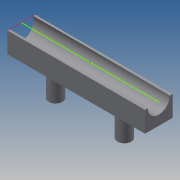
# Autodesk Inventor part: 滑軌2
Saved by Autodesk Inventor 2015 (Build 190159000, 159)
## iProperties
Created: 2018-01-06
Part Number: 滑軌2
Material: 一般
Document SubType Name: Modeling
Designer: user
Density: 1 g/cm^3
Appearance: 預設
Author: user
Autodesk Inventor part; units mm, degrees
ref_plane "YZ Plane" through (0, 0, 0) normal (1, 0, 0) x (0, 1, 0)
ref_plane "XZ Plane" through (0, 0, 0) normal (0, 1, 0) x (-1, 0, 0)
ref_plane "XY Plane" through (0, 0, 0) normal (0, 0, 1) x (1, 0, 0)
sketch "草圖1" plane through (0, 0, 0) normal (0, 0, 1) x (1, 0, 0)
  line L0 (-50, -10) -> (50, -10)
  line L1 (50, -10) -> (50, 10)
  line L2 (50, 10) -> (-50, 10)
  line L3 (-50, 10) -> (-50, -10)
  line L4 (-50, -10) -> (50, 10) construction
  line L5 (50, -10) -> (-50, 10) construction
  point P0 (0, 0)
  dimension "d0" = 20
  dimension "d1" = 100
  constraints: 12 end point, 2 midpoint, 2 parallel, 1 horizontal, 1 perpendicular
  measures "d0" distance of L0.end L1.end
  measures "d1" distance of L0.start L0.end
extrude "擠出1" add sketch "草圖1" along normal blind 15
sketch "草圖2" plane through (50, -10, 0) normal (1, 0, 0) x (0, 0, -1)
  circle A0 centre (-15, 10) radius 8
  line L0 (0, 0) -> (0, 20) projected
  point P0 (0, 10)
  dimension "d4" = 16
  dimension "d5" = 15
  constraints: 1 centre point
  measures "d4" diameter of A0
  measures "d5" distance from line of L0 A0.centre
sketch "草圖3" plane through (-50, -10, 0) normal (-1, 0, 0) x (0, 0, 1)
  circle A0 centre (12, 10) radius 9
  line L0 (0, 20) -> (0, 0) projected
  point P0 (0, 10)
  dimension "d6" = 18
  dimension "d7" = 12
  constraints: 1 centre point
  measures "d6" diameter of A0
  measures "d7" distance from line of L0 A0.centre
sketch "草圖4" plane through (0, 0, 15) normal (0, 0, 1) x (1, 0, 0)
  line L0 (49.8919, 0) -> (-50, 0)
  line L1 (-50, 10) -> (-50, -10) projected
  point P0 (0, 0)
  constraints: 2 end point, 1 midpoint
loft "斷面混成1" cut profiles "草圖3", "草圖2"
sketch "草圖5" plane through (0, 0, 0) normal (0, 0, -1) x (-1, 0, 0)
  circle A0 centre (25, 0) radius 5
  circle A1 centre (-25, 0) radius 5
  point P0 (0, 0)
  dimension "d12" = 10
  dimension "d13" = 10
  dimension "d14" = 50
  dimension "d15" = 25
  constraints: 2 centre point, 2 horizontal alignment
  measures "d12" diameter of A1
  measures "d13" diameter of A0
  measures "d14" distance of A1.centre A0.centre
  measures "d15" distance of point (0, 0) A1.centre
extrude "擠出2" add sketch "草圖5" along normal blind 20
